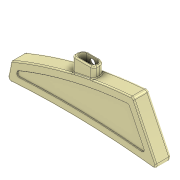
# Autodesk Inventor part: armsteun houder rechts
Saved by Autodesk Inventor 2020.3 (Build 243373000, 373)
## iProperties
Created: 2020-09-11
Part Number: armsteun houder rechts
Material: Stainless Steel
Document SubType Name: Modeling
Designer: Svend
Density: 8 g/cm^3
Appearance: Semi-Polished
Author: Svend
Autodesk Inventor part; units mm, degrees
ref_plane "YZ Plane" through (0, 0, 0) normal (1, 0, 0) x (0, 1, 0)
ref_plane "XY Plane" through (0, 0, 0) normal (0, 0, 1) x (1, 0, 0)
sketch "Sketch1" plane through (0, 0, 0) normal (0, 0, 1) x (1, 0, 0)
  arc A0 (0, 0) -> (-395, 10) centre (-247.8691, -1984.5808) ccw
  line L0 (0, 0) -> (-65.3835, 135)
  line L1 (0, 0) -> (0, 200) construction
  line L2 (-395, 10) -> (-385, 58.9898)
  arc A1 (-65.3835, 135) -> (-385, 58.9898) centre (3.0297, -862.6571) ccw
  dimension "d0" = 395
  dimension "d1" = 10
  dimension "d2" = 2000
  dimension "d3" = 200
  dimension "d5" = 150
  dimension "d6" = 135
  dimension "d7" = 50
  dimension "d8" = 10
  dimension "d9" = 1000
  constraints: 6 end point, 4 point on circle, 2 centre point, 1 coincident, 1 vertical
  measures "d0" horizontal distance of L2.start point (0, 0)
  measures "d1" vertical distance of L0.start L2.start
  measures "d2" radius of A0
  measures "d3" distance of L0.start L1.end
  measures "d5" distance of L0.start L0.end
  measures "d6" vertical distance of L0.start L0.end
  measures "d7" distance of L2.start L2.end
  measures "d8" horizontal distance of L2.start L2.end
  measures "d9" radius of A1
extrude "Extrusion1" add sketch "Sketch1" along normal blind 42
fillet "Fillet1" radius 8 4 edges at (-385, 58.9898, 21) (-395, 10, 21) (-65.3835, 135, 21) (0, 0, 21)
fillet "Fillet2" radius 8 8 edges at (-384.1832, 58.3296, 42) (-389.3691, 37.5857, 42) (-391.0737, 13.4591, 42) (-199.3066, 14.8295, 42) (-7.0707, 5.0677, 42) (-34.7051, 71.6572, 42) (-66.2255, 133.5656, 42) (-228.915, 110.0719, 42)
sketch "Sketch2" plane through (0, 0, 0) normal (0, 0, -1) x (-1, 0, 0)
  arc A0 (6.3894, 13.1924) -> (14.5228, 1.7599) centre (13.5894, 9.7053) ccw projected
  arc A1 (384.507, 10.7463) -> (14.5228, 1.7599) centre (247.8691, -1984.5808) ccw projected
  arc A2 (384.507, 10.7463) -> (392.8919, 20.3276) centre (385.0535, 18.7276) ccw projected
  line L0 (385.8463, 54.8437) -> (392.8919, 20.3276) projected
  arc A3 (385.8463, 54.8437) -> (381.0808, 60.63) centre (378.0079, 53.2437) ccw projected
  arc A4 (381.0808, 60.63) -> (70.8116, 134.6129) centre (-3.0297, -862.6571) ccw projected
  arc A5 (70.8116, 134.6129) -> (63.0209, 130.1219) centre (70.2209, 126.6348) ccw projected
  line L1 (6.3894, 13.1924) -> (63.0209, 130.1219) projected
  arc A6 (367.5281, 44.5843) -> (77.4508, 114.0327) centre (-3.0297, -862.6571) ccw
  line L2 (367.5281, 44.5843) -> (370.1552, 31.7144)
  arc A7 (370.1552, 31.7144) -> (33.871, 24.0518) centre (247.8691, -1984.5808) ccw
  line L3 (33.871, 24.0518) -> (77.4508, 114.0327)
  point P0 (0, 0)
  dimension "d14" = 20
  constraints: 4 end point, 4 point on circle, 2 centre point, 3 other
  measures "d14" distance between parallel lines of L1 L3
extrude "Extrusion2" cut sketch "Sketch2" against normal blind 2.5 contours L2 A7 L3 A6
fillet "Fillet3" radius 5 4 edges at (-370.1552, 31.7144, 1.25) (-367.5281, 44.5843, 1.25) (-77.4508, 114.0327, 1.25) (-33.871, 24.0518, 1.25)
fillet "Fillet4" radius 1 8 edges at (-38.1903, 27.0892, 0) (-56.8701, 71.5389, 0) (-77.9823, 113.1087, 0) (-225.5165, 90.3207, 0) (-367.0093, 44.1581, 0) (-368.4587, 40.0254, 0) (-367.7357, 33.8171, 0) (-203.0896, 34.9228, 0)
sketch "Sketch3" plane through (0, 0, 0) normal (0, 1, 0) x (-1, 0, 0)
  arc A0 (185.5149, 27) -> (185.5149, 7) centre (185.5149, 17) ccw
  arc A1 (213.5149, 7) -> (213.5149, 27) centre (213.5149, 17) ccw
  line L0 (185.5149, 7) -> (213.5149, 7)
  line L1 (213.5149, 27) -> (185.5149, 27)
  line L2 (14.5228, 0) -> (384.507, 0) projected
  line L3 (70.2209, 42) -> (378.0079, 42) construction
  line L4 (199.5149, 42) -> (199.5149, 0) construction
  arc A2 (185.5149, 32) -> (185.5149, 2) centre (185.5149, 17) ccw
  line L5 (185.5149, 32) -> (213.5149, 32)
  arc A3 (213.5149, 2) -> (213.5149, 32) centre (213.5149, 17) ccw
  line L6 (213.5149, 2) -> (185.5149, 2)
  line L7 (42.794, 2.5) -> (363.6683, 2.5) projected
  line L8 (228.5149, 17) -> (228.5149, 2.5)
  line L9 (170.5149, 2.5) -> (170.5149, 17.862)
  line L10 (228.5149, 2.5) -> (170.5149, 2.5)
  point P0 (0, 0)
  point P1 (199.5149, 7)
  point P2 (170.5149, 17)
  dimension "d19" = 20
  dimension "d20" = 28
  dimension "d21" = 7
  dimension "d22" = 5
  constraints: 17 end point, 10 point on circle, 5 tangent, 4 centre point, 3 point on line, 2 midpoint, 2 perpendicular, 1 equal radius, 1 horizontal, 1 horizontal alignment, 1 vertical alignment, 3 other
  measures "d19" diameter of A1
  measures "d20" distance of A0.centre A1.centre
  measures "d21" distance between parallel lines of L2 L0
  measures "d22" radial gap between concentric circles of A0 A2
extrude "Extrusion3" cut sketch "Sketch3" along normal through all contours L1 A1 L0 A0
ref_plane "Work Plane1" through (0, 108, 0) normal (0, 1, 0) x (-1, 0, 0)
sketch "Sketch4" plane through (0, 108, 0) normal (0, 1, 0) x (-1, 0, 0)
  line L0 (228.5149, 2.5) -> (170.5149, 2.5) projected
  line L1 (228.5149, 17) -> (228.5149, 2.5) projected
  arc A0 (213.5149, 2) -> (213.5149, 32) centre (213.5149, 17) ccw projected
  line L2 (185.5149, 32) -> (213.5149, 32) projected
  arc A1 (185.5149, 32) -> (185.5149, 2) centre (185.5149, 17) ccw projected
  line L3 (170.5149, 2.5) -> (170.5149, 17.862) projected
  spline S0 degree 7 poles (185.5149, 27) (184.6481, 27) (183.7899, 26.9123) (182.9543, 26.7402) (182.1545, 26.4902) (181.4023, 26.1726) (180.7069, 25.8006) (179.2526, 24.8577) (178.5264, 24.2534) (177.8936, 23.5966) (177.3502, 22.9012) (176.8917, 22.1775) (176.5139, 21.4329) (176.0119, 20.1616) (175.8451, 19.6432) (175.7125, 19.1195) (175.6136, 18.5921) (175.5478, 18.0622) (175.5149, 17.5312) (175.5149, 16.2584) (175.579, 15.517) (175.7073, 14.7791) (175.9005, 14.0476) (176.1605, 13.3265) (176.4899, 12.6206) (177.2054, 11.402) (177.5636, 10.8806) (177.9677, 10.3751) (178.4195, 9.8898) (178.9204, 9.4294) (179.4719, 9.0001) (180.7068, 8.1994) (181.4023, 7.8274) (182.1545, 7.5098) (182.9543, 7.2598) (183.7899, 7.0877) (184.6481, 7) (185.5149, 7) knots 0 0 0 0 0 0 0 0 0.157434 0.157434 0.157434 0.157434 0.157434 0.157434 0.362153 0.362153 0.362153 0.362153 0.362153 0.362153 0.499924 0.499924 0.499924 0.499924 0.499924 0.499924 0.692294 0.692294 0.692294 0.692294 0.692294 0.692294 0.842484 0.842484 0.842484 0.842484 0.842484 0.842484 1 1 1 1 1 1 1 1 projected
  line L4 (185.5149, 7) -> (213.5149, 7) projected
  spline S1 degree 7 poles (213.5149, 7) (214.3817, 7) (215.2399, 7.0877) (216.0756, 7.2599) (216.8754, 7.5099) (217.6276, 7.8275) (218.323, 8.1995) (219.7773, 9.1424) (220.5036, 9.7468) (221.1364, 10.4037) (221.6797, 11.0991) (222.1382, 11.8228) (222.5159, 12.5672) (223.0178, 13.8384) (223.1847, 14.3568) (223.3172, 14.8805) (223.4161, 15.4079) (223.482, 15.9378) (223.5149, 16.4689) (223.5149, 17.7416) (223.4507, 18.4829) (223.3225, 19.2208) (223.1293, 19.9522) (222.8693, 20.6734) (222.5399, 21.3794) (221.8243, 22.5979) (221.4662, 23.1193) (221.0622, 23.6247) (220.6104, 24.1101) (220.1095, 24.5705) (219.558, 24.9998) (218.323, 25.8005) (217.6276, 26.1725) (216.8754, 26.4901) (216.0756, 26.7401) (215.2399, 26.9123) (214.3817, 27) (213.5149, 27) knots 0 0 0 0 0 0 0 0 0.15738 0.15738 0.15738 0.15738 0.15738 0.15738 0.362112 0.362112 0.362112 0.362112 0.362112 0.362112 0.499925 0.499925 0.499925 0.499925 0.499925 0.499925 0.692347 0.692347 0.692347 0.692347 0.692347 0.692347 0.842538 0.842538 0.842538 0.842538 0.842538 0.842538 1 1 1 1 1 1 1 1 projected
  line L5 (213.5149, 27) -> (185.5149, 27) projected
  line L6 (384.507, 34) -> (14.5228, 34) projected
  line L7 (384.507, 0) -> (384.507, 34) projected
  line L8 (384.507, 0) -> (14.5228, 0) projected
  line L9 (14.5228, 34) -> (14.5228, 0) projected
  point P0 (0, 0)
  point P1 (170.5149, 17)
  constraints: 2 vertical alignment
extrude "Extrusion4" add sketch "Sketch4" along normal blind 40 contours L0 A0 L1 | L0 A1 L2 A0 | L0 L3 A1
fillet "Fillet5" radius 8 2 edges at (-228.5149, 129.0836, 2.5) (-170.5149, 135.0845, 2.5)
fillet "Fillet6" radius 2 8 edges at (-172.4476, 121.8264, 5.2857) (-170.5149, 122.1689, 13.75) (-174.0991, 121.5306, 26.7304) (-199.5356, 116.6117, 32) (-224.8677, 111.0281, 26.8038) (-228.5149, 110.1672, 13.75) (-226.5618, 110.63, 5.2622) (-199.5615, 116.6063, 2.5)
fillet "Fillet7" radius 3 8 edges at (-384.1832, 58.3296, 0) (-389.3691, 37.5857, 0) (-391.0737, 13.4591, 0) (-199.3066, 14.8295, 0) (-7.0707, 5.0677, 0) (-34.7051, 71.6572, 0) (-66.2255, 133.5656, 0) (-228.915, 110.0719, 0)
fillet "Fillet8" radius 3 8 edges at (-199.5149, 148, 32) (-174.9083, 148, 27.6066) (-170.5149, 148, 13.75) (-172.858, 148, 4.8431) (-199.5149, 148, 2.5) (-226.1717, 148, 4.8431) (-228.5149, 148, 13.75) (-224.1215, 148, 27.6066)
sketch "Sketch5" plane through (-213.5149, 145, 32) normal (0, 0, 1) x (1, 0, 0)
  circle A0 centre (14, -10) radius 7.5
  line L0 (28, 3) -> (0, 3) projected
  point P0 (213.5149, -145)
  point P1 (14, 3)
  dimension "d32" = 15
  dimension "d33" = 13
  constraints: 1 centre point, 1 midpoint, 1 vertical alignment
  measures "d32" diameter of A0
  measures "d33" distance from line of L0 A0.centre
extrude "Extrusion5" cut sketch "Sketch5" against normal blind 10
fillet "Fillet9" radius 1 1 edges at (-207.0149, 135, 32)
sketch "Sketch6" plane through (0, 0, 42) normal (0, 0, 1) x (1, 0, 0)
  line L0 (-185.5149, 14.447) -> (-185.5149, 148) projected
  line L1 (-213.5149, 15.1241) -> (-213.5149, 148) projected
  circle A0 centre (-199.5149, 135) radius 8.5 projected
  circle A1 centre (-199.5149, 135) radius 7.5 construction
  line L2 (-199.5149, 135) -> (-199.5149, 22.8369) construction
  arc A2 (-13.5894, 9.7053) -> (-385.0535, 18.7276) centre (-247.8691, -1984.5808) ccw construction
  ellipse E0 centre (-199.5149, 81) end of major axis (-169.5149, 81) minor radius 15
  line L3 (-175.5149, 14.11) -> (-175.5149, 148) projected
  point P0 (0, 0)
  dimension "d37" = 54
  dimension "d38" = 30
  dimension "d39" = 15
  constraints: 2 end point, 1 centre point, 1 point on circle, 1 point on line, 1 vertical, 1 other
  measures "d37" distance of A0.centre E0.centre
extrude "Extrusion6" cut sketch "Sketch6" against normal blind 12 contours E0 L1 L0 | L0 E0 L3 | E0 L1 | L3 E0
fillet "Fillet10" radius 4 1 edges at (-229.5149, 81, 42)
sketch "Sketch7" plane through (0, 0, 30) normal (0, 0, 1) x (1, 0, 0)
  ellipse E0 centre (-199.5149, 81) end of major axis (-169.5149, 81) minor radius 15 projected
  circle A0 centre (-199.5149, 81) radius 10
  point P0 (0, 0)
  dimension "d43" = 20
  constraints: 1 centre point, 1 coincident
  measures "d43" diameter of A0
extrude "Extrusion7" cut sketch "Sketch7" against normal up to next contours A0
fillet "Fillet11" radius 1 1 edges at (-209.5149, 81, 30)
fillet "Fillet12" radius 1 4 edges at (-199.5137, 14.8346, 7) (-223.5149, 15.2709, 17.002) (-199.5137, 14.8346, 27) (-175.5149, 14.11, 16.998)
mirror "Mirror1" about plane through (0, 0, 0) normal (0, 0, 1) remove original yes
body "Solid1"
